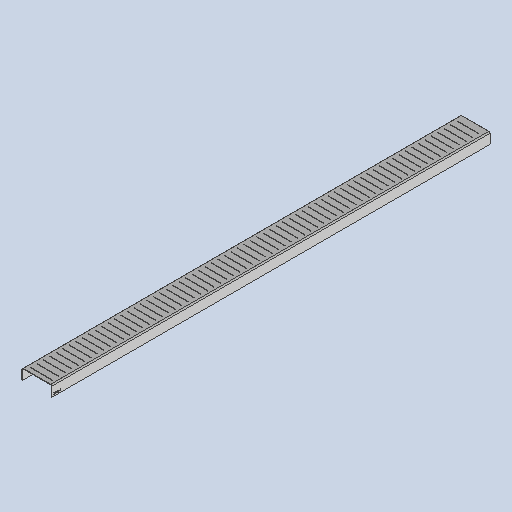
# Autodesk Inventor part: KND-5337 DrSysB roof 5 01
Saved by Autodesk Inventor 2026.2 (Build 302298000, 298)
## iProperties
Created: 2024-07-24
Part Number: KND-5337 DrSysB roof 5 01
Material: Stainless Steel
Document SubType Name: Sheet Metal
Designer: admin
Mass: 123.731 g
Surface Area: 420.588 cm^2
Volume: 15.4664 cm^3
Density: 8 g/cm^3
Flat Pattern Width: 6.88191 cm
Flat Pattern Length: 61 cm
Flat Pattern Area: 419.797 cm^2
Sheet Metal Rule: Default
Sheet Metal Width: 68,819 mm
Sheet Metal Length: 610,000 mm
Sheet Metal Area: 41979,660 mm^2
Appearance: Default
Author: admin
Autodesk Inventor part; units mm, degrees
ref_plane "YZ Plane" through (0, 0, 0) normal (1, 0, 0) x (0, 1, 0)
ref_plane "XZ Plane" through (0, 0, 0) normal (0, 1, 0) x (-1, 0, 0)
ref_plane "XY Plane" through (0, 0, 0) normal (0, 0, 1) x (1, 0, 0)
sketch "Sketch10" plane through (0, 0, 0) normal (0, 0, 1) x (1, 0, 0)
  line L0 (20, 0) -> (-20, 0)
  line L1 (-20, 0) -> (-20, 610)
  line L2 (-20, 610) -> (20, 610)
  line L3 (20, 610) -> (20, 0)
  point P0 (0, 0)
  point P1 (0, 0)
  dimension "d103" = 40
  dimension "d104" = 610
  measures "d103" distance of L1.end L2.end
  measures "d104" distance of L0.end L1.end
extrude "Plate2" add sketch "Sketch10" along normal blind 0.8
sketch "Sketch11" plane through (-20.8, 610, 0.8) normal (1, 0, 0) x (0, 1, 0)
  line L0 (-610, 0) -> (0, 0)
  line L1 (0, 0) -> (0, -15)
  line L2 (0, -15) -> (-610, -15)
  line L3 (-610, -15) -> (-610, 0)
  constraints: 8 end point
edge flange "Flange1" height 15 angle 90 thickness 0.8 bend radius 0.8 thickness toward (1, 0, 0) relief straight relief width 0.8 relief depth 0.4 corner gap 0.8 corner form 0 edges at (-20, 305, 0) (20, 305, 0) wall of the first edge with corners at (-20.8, 0, 0.8) (-20.8, 610, 0.8) (-20.8, 610, -14.2) (-20.8, 0, -14.2)
bend "Bend2"
corner "Corner2"
sketch "Sketch12" plane through (0, 0, 0.8) normal (0, 0, 1) x (1, 0, 0)
  line L0 (19.2, 0) -> (19.2, 610) construction
  line L1 (-19.2, 610) -> (19.2, 610) construction
  line L2 (-19.2, 610) -> (-19.2, 0) construction
  line L3 (19.2, 0) -> (-19.2, 0) construction
  line L4 (-15, 6.2) -> (15, 6.2) construction
  line L5 (-15, 6) -> (15, 6)
  line L6 (15, 6.4) -> (-15, 6.4)
  arc A0 (-15, 6.4) -> (-15, 6) centre (-15, 6.2) ccw
  arc A1 (15, 6) -> (15, 6.4) centre (15, 6.2) ccw
  line L7 (0, 6.2) -> (0, 0) construction
  point P0 (0, 0)
  dimension "d118" = 0.4
  dimension "d119" = 6
  dimension "d120" = 30
  constraints: 10 end point, 4 point on circle, 4 tangent, 2 centre point, 2 midpoint, 1 horizontal, 1 parallel, 1 vertical, 1 vertical alignment
  measures "d118" diameter of A1
  measures "d119" distance between parallel lines of L3 L5
  measures "d120" distance of L4.start L4.end
extrude "Extrusion5" cut sketch "Sketch12" against normal blind 5
sketch "Sketch13" plane through (0, 0, 0) normal (1, 0, 0) x (0, 1, 0)
  line L0 (6.4, 0.8) -> (6.4, 0) projected
  line L1 (6, 0.8) -> (6, 0) projected
  line L2 (6.15, -1.2) -> (6.15, -8.2) construction
  line L3 (6.4, -1.2) -> (6.4, -8.2)
  line L4 (5.9, -8.2) -> (5.9, -1.2)
  arc A0 (6.4, -1.2) -> (5.9, -1.2) centre (6.15, -1.2) ccw
  arc A1 (5.9, -8.2) -> (6.4, -8.2) centre (6.15, -8.2) ccw
  point P0 (0, 0)
  point P1 (13, -4.2)
  point P2 (13.3, -4.2)
  point P3 (6.15, -4.7)
  dimension "d129" = 7
  constraints: 8 end point, 4 point on circle, 4 tangent, 2 centre point, 1 collinear, 1 midpoint, 1 parallel, 1 vertical
  measures "d129" distance of L2.start L2.end
extrude "Extrusion6" [suppressed]
pattern_linear "Rectangular Pattern3" count 67 spacing 9 along (0, 1, 0) of "Extrusion5"
sketch "Sketch14" plane through (20.8, 0, -14.2) normal (1, 0, 0) x (0, 0, -1)
  line L0 (-4.8646, 1.9039) -> (-4.8646, 27.6803) construction
  line L1 (-4.8646, 27.6803) -> (-1.2058, 27.6803) construction
  line L2 (-1.2058, 27.6803) -> (-1.2058, 1.9039) construction
  line L3 (-1.2058, 1.9039) -> (-4.8646, 1.9039) construction
  point P0 (-14.2, 0)
  point P1 (-0.4628, -6.744)
  dimension "d134" = 9
  dimension "Filter_cm" = 260
  constraints: 2 other
mark "Mark4"
derived "KND-1401 DrSysB DIMentions 01.ipt"
equation "\"Filter_cm\" = 260"
equation "\"BendRadius\" = Thickness"
equation "\"BendReliefWidth\" = Thickness"
equation "\"BendReliefDepth\" = 0.5 * Thickness"
equation "\"CornerReliefSize\" = 4 * Thickness"
equation "\"MinimumRemnant\" = 2 * Thickness"
equation "\"TransitionRadius\" = BendRadius"
equation "\"JacobiRadiusSize\" = BendRadius"
equation "\"GapSize\" = Thickness"
equation "\"grat_thick\" = 0.2"
equation "\"grat_indet_X\" = 5"
equation "\"grat_indet_Y\" = 0.5"
equation "\"grat_number\" = 43.571429"
equation "\"grat_step\" = 7"
equation "\"BEAM_2_lenth\" = 335"
equation "\"BEAM_2_angle\" = 6deg"
equation "\"Thickness\" = 0.8"
body "Solid3"
